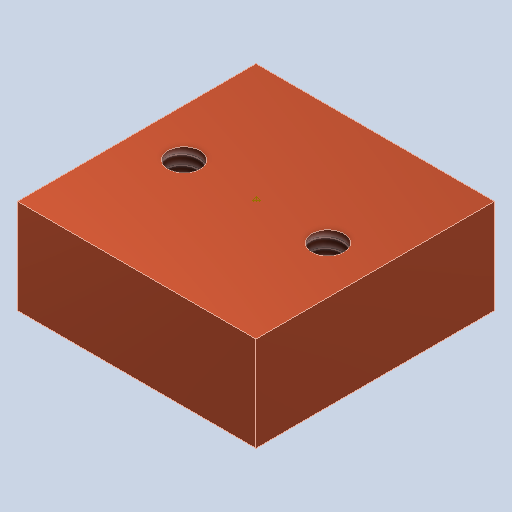
# Autodesk Inventor part: bottom_cu_block
Saved by Autodesk Inventor 2024.2 (Build 282272000, 272)
## iProperties
Created: 2023-03-15
Part Number: bottom_cu_block
Material: Copper
Document SubType Name: Modeling
Designer: warke
Density: 8.94 g/cm^3
Appearance: Copper - Satin
Author: warke
Autodesk Inventor part; units mm, degrees
ref_plane "YZ Plane" through (0, 0, 0) normal (1, 0, 0) x (0, 1, 0)
ref_plane "XZ Plane" through (0, 0, 0) normal (0, 1, 0) x (-1, 0, 0)
ref_plane "XY Plane" through (0, 0, 0) normal (0, 0, 1) x (1, 0, 0)
sketch "Sketch1" plane through (0, 0, 0) normal (0, 1, 0) x (-1, 0, 0)
  line L0 (8, 8) -> (-8, 8)
  line L1 (-8, 8) -> (-8, -8)
  line L2 (-8, -8) -> (8, -8)
  line L3 (8, -8) -> (8, 8)
  line L4 (8, 8) -> (-8, -8) construction
  line L5 (-8, 8) -> (8, -8) construction
  point P0 (0, 0)
  dimension "d0" = 16
  dimension "d1" = 16
  constraints: 12 end point, 2 midpoint, 2 parallel, 1 horizontal, 1 perpendicular
  measures "d0" distance of L2.end L1.end
  measures "d1" distance of L1.end L0.end
extrude "Extrusion1" add sketch "Sketch1" along normal blind 6.35
sketch "Sketch2" plane through (0, 6.35, 0) normal (0, 1, 0) x (1, 0, 0)
  line L0 (-8, 8) -> (-8, -8) projected
  line L1 (8, -8) -> (8, 8) projected
  point P0 (0, 0)
  point P1 (-4.825, 0)
  point P2 (4.825, 0)
hole "Hole1" at (-4.825, 6.35, 0) at (4.825, 6.35, 0) direction (0, -1, 0) diameter 2.1565 depth 4.29 thread size "4-40 UNC" class "2B" standard "ANSI Unified Screw Threads"
sketch "Sketch3" plane through (8, 0, -8) normal (0, 0, -1) x (-1, 0, 0)
  point P0 (8, 0)
body "Solid1"
